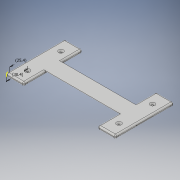
# Autodesk Inventor part: TapeMeasureBracketBase
Saved by Autodesk Inventor 2019 (Build 230136000, 136)
## iProperties
Created: 2018-11-04
Part Number: TapeMeasureBracketBase
Material: Generic
Document SubType Name: Modeling
Designer: mrhftc
Density: 1 g/cm^3
Appearance: Default
Author: mrhftc
Autodesk Inventor part; units mm, degrees
ref_plane "YZ Plane" through (0, 0, 0) normal (1, 0, 0) x (0, 1, 0)
ref_plane "XZ Plane" through (0, 0, 0) normal (0, 1, 0) x (-1, 0, 0)
ref_plane "XY Plane" through (0, 0, 0) normal (0, 0, 1) x (1, 0, 0)
sketch "Sketch1" plane through (0, 0, 0) normal (0, 1, 0) x (-1, 0, 0)
  line L0 (-77.5, -41.5) -> (77.5, -41.5)
  line L1 (77.5, -41.5) -> (77.5, 41.5)
  line L2 (77.5, 41.5) -> (-77.5, 41.5)
  line L3 (-77.5, 41.5) -> (-77.5, -41.5)
  line L4 (-77.5, -41.5) -> (77.5, 41.5) construction
  line L5 (77.5, -41.5) -> (-77.5, 41.5) construction
  point P0 (0, 0)
  dimension "d1" = 83
  dimension "d4" = 155
  constraints: 12 end point, 2 midpoint, 2 parallel, 1 horizontal, 1 perpendicular
  measures "d1" distance of L0.end L1.end
  measures "d4" distance of L0.start L0.end
extrude "Extrusion1" add sketch "Sketch1" along normal blind 5
sketch "Sketch2" plane through (-77.5, 0, -41.5) normal (-1, 0, 0) x (0, 0, 1)
  line L0 (78, 2) -> (52.6, 2)
  line L1 (52.6, 2) -> (52.6, 3)
  line L2 (52.6, 3) -> (78, 3)
  line L3 (78, 3) -> (78, 2)
  line L4 (83, 0) -> (83, 5) projected
  line L5 (41.5, 0) -> (41.5, 5)
  line L6 (0, 0) -> (83, 0) projected
  line L7 (0, 5) -> (83, 5) projected
  line L8 (5, 2) -> (30.4, 2)
  line L9 (30.4, 2) -> (30.4, 3)
  line L10 (30.4, 3) -> (5, 3)
  line L11 (5, 3) -> (5, 2)
  line L12 (0, 0) -> (0, 5) projected
  dimension "d7" = 25.4
  dimension "d8" = 1
  dimension "d9" = 5
  dimension "d10" = 2
  dimension "d11" = 2
  dimension "d12" = 5
  constraints: 18 end point, 4 symmetric about line, 2 parallel, 1 horizontal, 1 perpendicular, 1 vertical
  measures "d7" distance of L0.start L0.end
  measures "d8" distance of L2.end L0.start
  measures "d9" distance between parallel lines of L3 L4
  measures "d10" distance between parallel lines of L0 L6
  measures "d11" distance between parallel lines of L7 L2
  measures "d12" distance from line of L8.start L12
extrude "Extrusion2" cut sketch "Sketch2" against normal blind 165.1 contours L0 L1 L2 L3 | L11 L10 L9 L8
sketch "Sketch3" plane through (-77.5, 0, 41.5) normal (0, 0, 1) x (1, 0, 0)
  line L0 (155, 0) -> (0, 0) projected
  line L1 (155, 5) -> (0, 5) projected
  line L2 (130, 0) -> (25, 0)
  line L3 (25, 0) -> (25, 5)
  line L4 (25, 5) -> (130, 5)
  line L5 (130, 5) -> (130, 0)
  line L6 (0, 0) -> (0, 5) projected
  line L7 (155, 0) -> (155, 5) projected
  point P0 (77.5, 0)
  dimension "d15" = 155
  dimension "d16" = 105
  dimension "d17" = 25
  constraints: 8 end point, 2 parallel, 2 point on line, 1 horizontal, 1 perpendicular
  measures "d15" distance between parallel lines of L6 L7
  measures "d16" distance between parallel lines of L3 L5
  measures "d17" distance between parallel lines of L7 L5
sketch "Sketch4" plane through (-77.5, 0, -41.5) normal (-1, 0, 0) x (0, 0, 1)
  line L0 (52.6, 2) -> (52.6, 3) projected
  line L1 (83, 0) -> (83, 5) projected
  point P0 (41.5, 0)
  dimension "d18" = 30.4
  measures "d18" distance between parallel lines of L0 L1
extrude "Extrusion3" cut sketch "Sketch3" against normal blind 30.4 contours L0 L3 L1 L5
sketch "Sketch5" plane through (0, 0, 0) normal (0, -1, 0) x (1, 0, 0)
  point P0 (0, 0)
mirror "Mirror1" about plane through (0, 0, 0) normal (0, 0, 1) of "Extrusion3"
sketch "Sketch6" plane through (0, 0, 0) normal (0, -1, 0) x (1, 0, 0)
  line L0 (-52.5, -11.1) -> (52.5, -11.1) projected
  line L1 (-52.5, 11.1) -> (52.5, 11.1)
  line L2 (52.5, 11.1) -> (52.5, -11.1)
  line L3 (52.5, -11.1) -> (-52.5, -11.1)
  line L4 (-52.5, -11.1) -> (-52.5, 11.1)
  point P0 (0, 0)
  constraints: 8 end point, 2 parallel, 1 horizontal, 1 perpendicular
extrude "Extrusion4" cut sketch "Sketch6" against normal blind 3
fillet "Fillet1" radius 2 18 edges at (77.5, 2.5, -41.5) (77.5, 0, 0) (52.5, 0, 0) (52.5, 2.5, -41.5) (0, 3, -11.1) (-52.5, 0, 0) (-77.5, 0, 0) (-65, 0, -41.5) (-52.5, 2.5, -41.5) (-77.5, 2.5, -41.5) (65, 0, -41.5) (77.5, 2.5, 41.5) (65, 0, 41.5) (52.5, 2.5, 41.5) (0, 3, 11.1) (-65, 0, 41.5) (-77.5, 2.5, 41.5) (-52.5, 2.5, 41.5)
sketch "Sketch7" plane through (0, 0, 0) normal (0, -1, 0) x (1, 0, 0)
  point P0 (0, 0)
sketch "Sketch8" plane through (-77.5, 3, -36.5) normal (-1, 0, 0) x (0, 0, 1)
  point P0 (36.5, -3)
sketch "Sketch9" plane through (-77.5, 3, -36.5) normal (-1, 0, 0) x (0, 0, 1)
  line L0 (73, 0) -> (73, -1) projected
  line L1 (47.6, -1) -> (47.6, 0) projected
  point P0 (36.5, -3)
  dimension "d24" = 25.4
  measures "d24" distance between parallel lines of L0 L1
sketch "Sketch10" plane through (0, 0, 0) normal (0, -1, 0) x (1, 0, 0)
  point P0 (0, 0)
sketch "Sketch11" plane through (-77.5, 3, -36.5) normal (-1, 0, 0) x (0, 0, 1)
  line L0 (73, 0) -> (73, -1) projected
  line L1 (78, -1) -> (78, 2) projected
  line L2 (76, 2) -> (76, -1) projected
  line L3 (47.6, -1) -> (47.6, 0) projected
  point P0 (36.5, -3)
sketch "Sketch12" plane through (0, 0, 0) normal (0, -1, 0) x (1, 0, 0)
  circle A0 centre (-65, 23.8) radius 1.5
  line L0 (-75.5, 39.5) -> (-54.5, 39.5) projected
  line L1 (-75.5, -39.5) -> (-75.5, 39.5) projected
  line L2 (-54.5, 39.5) -> (-54.5, -39.5) projected
  line L3 (-54.5, 0) -> (-77.3446, 0)
  circle A1 centre (-65, -23.8) radius 1.5
  line L4 (-54.5, -39.5) -> (-75.5, -39.5) projected
  line L5 (52.5, -9.1) -> (-52.5, -9.1) projected
  line L6 (0, -9.1) -> (0, 8.7202)
  circle A2 centre (65, 23.8) radius 1.5
  circle A3 centre (65, -23.8) radius 1.5
  line L7 (75.5, 39.5) -> (75.5, -39.5) projected
  line L8 (75.5, -39.5) -> (54.5, -39.5) projected
  line L9 (54.5, -39.5) -> (54.5, 39.5) projected
  line L10 (54.5, 39.5) -> (75.5, 39.5) projected
  point P0 (0, 0)
  point P1 (-65, 0)
  dimension "d28" = 3
  dimension "d29" = 15.7
  dimension "d30" = 21
  dimension "d31" = 10.5
  dimension "d32" = 10.5
  dimension "d33" = 23.8
  dimension "d34" = 15.7
  dimension "d35" = 23.8
  dimension "d36" = 10.5
  dimension "d37" = 15.7
  dimension "d38" = 10.5
  dimension "d39" = 15.7
  constraints: 4 centre point, 4 end point, 3 symmetric about line, 2 midpoint, 1 perpendicular, 1 vertical, 3 other
  measures "d28" diameter of A0
  measures "d29" distance from line of L0 A0.centre
  measures "d30" distance between parallel lines of L1 L2
  measures "d31" distance from line of L2 A0.centre
  measures "d32" distance from line of L1 A0.centre
  measures "d33" distance of A0.centre point (-65, 0)
  measures "d34" distance from line of A1.centre L4
  measures "d35" distance of point (-65, 0) A1.centre
  measures "d36" distance from line of A3.centre L7
  measures "d37" distance from line of L8 A3.centre
  measures "d38" distance from line of L9 A2.centre
  measures "d39" distance from line of L10 A2.centre
extrude "Extrusion5" cut sketch "Sketch12" against normal through all contours A0 | A1 | A2 | A3
fillet "Fillet2" radius 2 18 edges at (77.5, 5, 0) (76.9142, 5, -40.9142) (65, 5, -41.5) (53.0858, 5, -40.9142) (52.5, 5, -25.3001) (76.9142, 5, 40.9142) (65, 5, 41.5) (53.0858, 5, 40.9142) (52.5, 5, 25.3) (-53.0858, 5, -40.9142) (-65, 5, -41.5) (-76.9142, 5, -40.9142) (-77.5, 5, 0) (-76.9142, 5, 40.9142) (-65, 5, 41.5) (-53.0858, 5, 40.9142) (-52.5, 5, 25.3) (-52.5, 5, -25.3)
fillet "Fillet3" radius 2 1 edges at (63.5, 0, -23.8)
fillet "Fillet4" radius 2 3 edges at (63.5, 0, 23.8) (-66.5, 0, 23.8) (-66.5, 0, -23.8)
fillet "Fillet5" radius 2 1 edges at (63.5, 5, -23.8)
fillet "Fillet6" radius 2 3 edges at (63.5, 5, 23.8) (-66.5, 5, 23.8) (-66.5, 5, -23.8)
body "Solid1"
